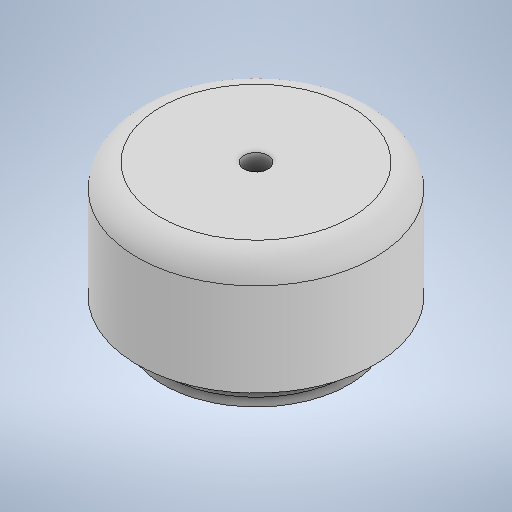
# Autodesk Inventor part: Water_Sensor_Cap
Saved by Autodesk Inventor 2025 (Build 290162000, 162)
## iProperties
Created: 2024-06-19
Part Number: Water_Sensor_Cap
Material: Generic
Document SubType Name: Modeling
Designer: track
Density: 1 g/cm^3
Appearance: Default
Mass: 56.6087 g
Surface Area: 245.5 cm^2
Volume: 56.6087 cm^3
Author: track
## iProperties of the stored document Water_Sensor_Cap_3DPrint.ipt
Created: 2024-06-19
Part Number: Water_Sensor_Cap_3DPrint
Material: Generic
Document SubType Name: Modeling
Designer: track
Density: 1 g/cm^3
Appearance: Default
Author: track
Autodesk Inventor part; units mm, degrees
ref_plane "YZ Plane" through (0, 0, 0) normal (1, 0, 0) x (0, 1, 0)
ref_plane "XZ Plane" through (0, 0, 0) normal (0, 1, 0) x (-1, 0, 0)
ref_plane "XY Plane" through (0, 0, 0) normal (0, 0, 1) x (1, 0, 0)
sketch "Sketch1" plane through (0, 0, 0) normal (0, 1, 0) x (-1, 0, 0)
  circle A0 centre (0, 0) radius 30.48
  circle A1 centre (0, 0) radius 32.48
  dimension "d0" = 60.96
  dimension "d2" = 2
  constraints: 2 centre point, 2 coincident
  measures "d0" diameter of A0
  measures "d2" radial gap between concentric circles of A1 A0
extrude "Extrusion1" add sketch "Sketch1" along normal blind 19.05
sketch "Sketch2" plane through (0, 19.05, 0) normal (0, 1, 0) x (1, 0, 0)
  circle A0 centre (0, 0) radius 32.48
  circle A1 centre (0, 0) radius 32.48 projected
  constraints: 1 centre point, 1 coincident, 1 concentric
extrude "Extrusion2" add sketch "Sketch2" along normal blind 12.7
fillet "Fillet1" radius 6.35 1 edges at (-32.48, 31.75, 0)
sketch "Sketch6" plane through (0, 31.75, 0) normal (0, 1, 0) x (1, 0, 0)
  circle A0 centre (0, 0) radius 3.302
  dimension "d15" = 6.604
  constraints: 1 centre point, 1 coincident
  measures "d15" diameter of A0
extrude "Extrusion5" cut sketch "Sketch6" against normal up to surface (12.7 mm away)
sketch "Sketch10" plane through (0, 0, 0) normal (0, 0, 1) x (1, 0, 0)
  line L0 (-17.78, 19.05) -> (-17.78, -12.7)
  line L1 (-17.78, -12.7) -> (-25.4, -12.7)
  line L2 (-25.4, -12.7) -> (-25.4, 19.05)
  line L3 (-17.78, 19.05) -> (-25.4, 19.05)
  line L4 (-26.13, 31.75) -> (26.13, 31.75) projected
  line L5 (0, 31.75) -> (0, 0)
  line L6 (32.48, 0) -> (-32.48, 0) projected
  line L7 (-30.48, 0) -> (-30.48, 19.05)
  line L8 (-17.78, -12.7) -> (-25.4, -8.3006)
  line L9 (-30.48, 19.05) -> (30.48, 19.05) projected
  point P0 (-30.48, 0)
  point P1 (-25.4, 19.05)
  dimension "d29" = 7.62
  dimension "d33" = 30
  dimension "d42" = 25.4
  dimension "d89" = 31.75
  constraints: 12 end point, 3 perpendicular, 2 point on line, 2 vertical, 1 horizontal, 1 midpoint, 3 other
  measures "d29" distance between parallel lines of L0 L2
  measures "d33" angle of L1 L8
  measures "d42" distance between parallel lines of L5 L2
  measures "d89" distance between parallel lines of L9 L1
revolve "Revolution2" add sketch "Sketch10" angle 360 about axis through (0, 31.75, 0) along (0, -1, 0) contours L0 L6 L2 L3 | L0 L8 L2 L6
sketch "Sketch11" plane through (0, 0, 0) normal (0, 0, 1) x (1, 0, 0)
  line L0 (25.4, -7.0306) -> (25.4, 25.4)
  circle A0 centre (26.3462, -3.81) radius 2.3813
  circle A1 centre (26.3462, 2.54) radius 2.3813
  line L1 (0, -11.43) -> (0, 31.75)
  line L2 (-26.13, 31.75) -> (26.13, 31.75) projected
  line L3 (26.3462, 2.54) -> (26.3462, -3.81)
  line L4 (30.48, 19.05) -> (30.48, 0) projected
  line L5 (30.48, 0) -> (29.972, 19.05)
  line L6 (29.972, 19.05) -> (29.972, 0) projected
  line L7 (-25.4, -5.08) -> (25.4, -5.08) projected
  line L8 (-17.78, -12.7) -> (17.78, -12.7) projected
  point P0 (0, 0)
  point P1 (25.4, -8.3006)
  point P2 (27.772, -0.6806)
  point P3 (17.78, -12.7)
  dimension "d36" = 6.35
  dimension "d37" = 4.7625
  dimension "d38" = 4.7625
  dimension "d43" = 26.3462
  dimension "d91" = 8.89
  constraints: 8 end point, 2 centre point, 2 vertical, 1 midpoint, 1 point on line, 4 other
  measures "d36" distance of L3.end L3.start
  measures "d37" diameter of A1
  measures "d38" diameter of A0
  measures "d43" distance between parallel lines of L1 L3
revolve "Revolution3" cut sketch "Sketch11" angle 360 about axis through (0, -11.43, 0) along (0, 1, 0) contours A0 L7 L0 | L0 A0 | L7 A0 L0 | A1 L0 | L0 A1
body "Solid1"
